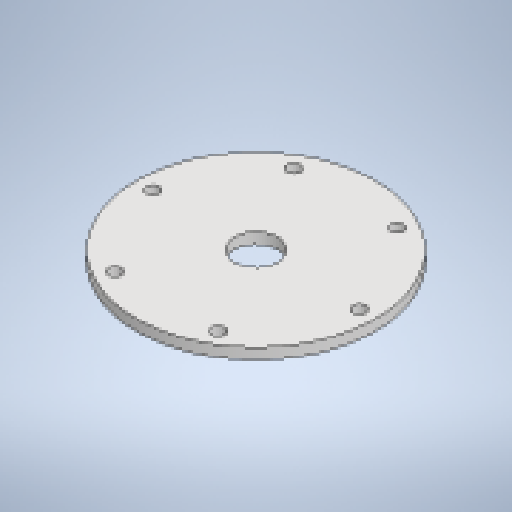
# Autodesk Inventor part: NVPH-343 cup head flange
Saved by Autodesk Inventor 2025 (Build 290162010, 162A)
## iProperties
Created: 2024-12-03
Part Number: NVPH-343 cup head flange
Material: Generic
Document SubType Name: Sheet Metal
Designer: user
Density: 1 g/cm^3
Flat Pattern Width: 22 cm
Flat Pattern Length: 22 cm
Flat Pattern Area: 484 cm^2
Sheet Metal Rule: Default_mm
Sheet Metal Width: 220,000 mm
Sheet Metal Length: 220,000 mm
Sheet Metal Area: 48400,000 mm^2
Appearance: Default
Mass: 294.807 g
Surface Area: 687.632 cm^2
Volume: 294.807 cm^3
Author: user
Autodesk Inventor part; units mm, degrees
ref_plane "YZ Plane" through (0, 0, 0) normal (1, 0, 0) x (0, 1, 0)
ref_plane "XZ Plane" through (0, 0, 0) normal (0, 1, 0) x (-1, 0, 0)
ref_plane "XY Plane" through (0, 0, 0) normal (0, 0, 1) x (1, 0, 0)
sketch "Sketch1" plane through (0, 0, 0) normal (0, 0, 1) x (1, 0, 0)
  circle A0 centre (0, 0) radius 20
  circle A1 centre (0, 0) radius 110
  dimension "d0" = 40
  dimension "d1" = 220
  constraints: 2 centre point, 2 coincident
  measures "d0" diameter of A0
  measures "d1" diameter of A1
extrude "Extrusion1" add sketch "Sketch1" against normal blind 10
sketch "Sketch3" plane through (0, 0, 0) normal (0, 0, 1) x (1, 0, 0)
  circle A0 centre (95, 0) radius 6
  circle A1 centre (0, 0) radius 95 construction
  circle A2 centre (0, 0) radius 110 projected
  dimension "d5" = 12
  dimension "d12" = 15
  constraints: 2 horizontal alignment, 1 centre point, 1 coincident, 2 other
  measures "d5" diameter of A0
extrude "Cut1" cut sketch "Sketch3" against normal blind 10 contours A0
pattern_circular "Circular Pattern1" count 6 over 360 about axis through (0, 0, 0) along (0, 0, -1) of "Cut1"
equation "\"d7\" = Thickness"
equation "\"BendReliefDepth\" = 0.5 * Thickness"
equation "\"Thickness\" = 10"
body "Solid1"
